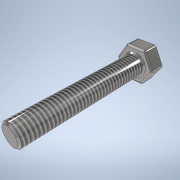
# Autodesk Inventor part: Болт М5х30
Saved by Autodesk Inventor 2021.1 (Build 251245010, 245A)
## iProperties
Created: 2025-12-08
Part Number: Болт М5х30
Material: Типовые
Document SubType Name: Modeling
Designer: Андрей Тарасов
Density: 1 g/cm^3
Appearance: По умолчанию
Author: Андрей Тарасов
Autodesk Inventor part; units mm, degrees
ref_plane "YZ Plane" through (0, 0, 0) normal (1, 0, 0) x (0, 1, 0)
ref_plane "XZ Plane" through (0, 0, 0) normal (0, 1, 0) x (-1, 0, 0)
ref_plane "XY Plane" through (0, 0, 0) normal (0, 0, 1) x (1, 0, 0)
sketch "Эскиз1" plane through (0, 0, 0) normal (0, 0, 1) x (1, 0, 0)
  line L0 (-2.3094, 4) -> (2.3094, 4)
  line L1 (2.3094, 4) -> (4.6188, 0)
  line L2 (4.6188, 0) -> (2.3094, -4)
  line L3 (2.3094, -4) -> (-2.3094, -4)
  line L4 (-2.3094, -4) -> (-4.6188, 0)
  line L5 (-4.6188, 0) -> (-2.3094, 4)
  point P0 (0, 0)
  point P1 (0, 0)
  dimension "d0" = 8
  constraints: 12 end point, 1 coincident, 1 horizontal, 13 other
  measures "d0" distance between parallel lines of L0 L3
extrude "Выдавливание1" add sketch "Эскиз1" along normal blind 4
sketch "Эскиз2" plane through (0, 0, 4) normal (0, 0, 1) x (1, 0, 0)
  circle A0 centre (0, 0) radius 2.5
  dimension "d3" = 5
  constraints: 1 centre point, 1 coincident
  measures "d3" diameter of A0
extrude "Выдавливание2" add sketch "Эскиз2" along normal blind 30
fillet "Сопряжение1" radius 0.6 6 edges at (-2.3094, -4, 2) (2.3094, -4, 2) (4.6188, 0, 2) (2.3094, 4, 2) (-2.3094, 4, 2) (-4.6188, 0, 2)
chamfer "Фаска1" distance 0.4 angle 45 26 edges at (3.4641, 2, 4) (2.263, 3.9196, 4) (0, 4, 4) (-2.263, 3.9196, 4) (-3.4641, 2, 4) (-4.526, 0, 4) (-3.4641, -2, 4) (-2.263, -3.9196, 4) (0, -4, 4) (2.263, -3.9196, 4) (3.4641, -2, 4) (4.526, 0, 4) (-3.4641, 2, 0) (-4.526, 0, 0) (-3.4641, -2, 0) (-2.263, -3.9196, 0) (0, -4, 0) (2.263, -3.9196, 0) (3.4641, -2, 0) (4.526, 0, 0) (3.4641, 2, 0) (2.263, 3.9196, 0) (0, 4, 0) (-2.263, 3.9196, 0) (-2.5, 0, 34) (-2.5, 0, 4)
thread "Резьба1" size "M5x0.8" class "6g" standard "ANSI Metric M Profile" full length
